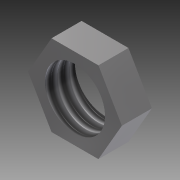
# Autodesk Inventor part: LCD Nut
Saved by Autodesk Inventor 2015 (Build 190159000, 159)
## iProperties
Created: 2015-11-02
Part Number: LCD Nut
Material: Stainless Steel
Document SubType Name: Modeling
Designer: James
Density: 8 g/cm^3
Appearance: Semi-Polished
Author: James
Autodesk Inventor part; units mm, degrees
ref_plane "YZ Plane" through (0, 0, 0) normal (1, 0, 0) x (0, 1, 0)
ref_plane "XZ Plane" through (0, 0, 0) normal (0, 1, 0) x (-1, 0, 0)
ref_plane "XY Plane" through (0, 0, 0) normal (0, 0, 1) x (1, 0, 0)
sketch "Sketch1" plane through (0, 0, 0) normal (0, 1, 0) x (-1, 0, 0)
  circle A0 centre (0, 0) radius 1
  line L0 (1.5588, 0) -> (0.7794, -1.35)
  line L1 (0.7794, -1.35) -> (-0.7794, -1.35)
  line L2 (-0.7794, -1.35) -> (-1.5588, 0)
  line L3 (-1.5588, 0) -> (-0.7794, 1.35)
  line L4 (-0.7794, 1.35) -> (0.7794, 1.35)
  line L5 (0.7794, 1.35) -> (1.5588, 0)
  dimension "d0" = 2
  dimension "d1" = 2.7
  constraints: 12 end point, 2 coincident, 1 centre point, 13 other
  measures "d0" diameter of A0
  measures "d1" distance between parallel lines of L1 L4
extrude "Extrusion1" add sketch "Sketch1" along normal blind 1
thread "Thread1" size "M2x0.4" class "6H" standard "ANSI Metric M Profile" full length
body "Solid1"
